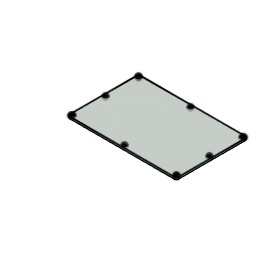
Lid - Compact (Autodesk Fusion 360 design; units mm, degrees)
Autodesk Fusion 360 part; units mm, degrees
sketch "Sketch1" plane through (0, 0, 123.8) normal (0, 0, 1) x (-1, 0, 0)
  line L0 (68.8, -91.5) -> (68.8, -99.5)
  line L1 (68.8, -99.5) -> (86.5, -99.5)
  arc A0 (86.5, -99.5) -> (89.5, -96.5) centre (86.5, -96.5) ccw
  line L2 (89.5, -96.5) -> (89.5, 14.2937)
  arc A1 (89.5, 14.2937) -> (86.5, 17.2937) centre (86.5, 14.2937) ccw
  line L3 (86.5, 17.2937) -> (-86.5, 17.2937)
  arc A2 (-86.5, 17.2937) -> (-89.5, 14.2937) centre (-86.5, 14.2937) ccw
  line L4 (-89.5, 14.2937) -> (-89.5, -96.5)
  arc A3 (-89.5, -96.5) -> (-86.5, -99.5) centre (-86.5, -96.5) ccw
  line L5 (-86.5, -99.5) -> (8.2, -99.5)
  line L6 (8.2, -99.5) -> (8.2, -91.5)
  line L7 (8.2, -91.5) -> (-71.5, -91.5)
  arc A4 (-81.5, -81.5) -> (-71.5, -91.5) centre (-71.5, -81.5) ccw
  line L8 (-81.5, -81.5) -> (-81.5, -0.7063)
  arc A5 (-71.5, 9.2937) -> (-81.5, -0.7063) centre (-71.5, -0.7063) ccw
  line L9 (-71.5, 9.2937) -> (71.5, 9.2937)
  arc A6 (81.5, -0.7063) -> (71.5, 9.2937) centre (71.5, -0.7063) ccw
  line L10 (81.5, -0.7063) -> (81.5, -81.5)
  arc A7 (71.5, -91.5) -> (81.5, -81.5) centre (71.5, -81.5) ccw
  line L11 (71.5, -91.5) -> (68.8, -91.5)
  circle A8 centre (-85.5, -95.5) radius 1.9
  circle A9 centre (85.5, 13.2937) radius 1.9
  circle A10 centre (85.5, -95.5) radius 1.9
  circle A11 centre (0, 13.2937) radius 1.9
  circle A12 centre (-85.5, -41.1031) radius 1.9
  circle A13 centre (-85.5, 13.2937) radius 1.9
  circle A14 centre (85.5, -41.1031) radius 1.9
  circle A15 centre (0, -95.5) radius 1.9
  line L12 (68.8, -99.5) -> (8.2, -99.5)
  constraint coincident L0.end L1.start
  constraint coincident L5.end L6.start
extrude "Extrude1" add sketch "Sketch1" along normal blind 3
sketch "Sketch2" plane through (0, 0, 126.8) normal (0, 0, 1) x (-1, 0, 0)
  circle A0 centre (-85.5, 13.2937) radius 1.9
  circle A1 centre (85.5, 13.2937) radius 1.9
  circle A2 centre (-85.5, -41.1031) radius 1.9
  circle A3 centre (85.5, -41.1031) radius 1.9
  circle A4 centre (0, 13.2937) radius 1.9
  circle A5 centre (-85.5, -95.5) radius 1.9
  circle A6 centre (0, -95.5) radius 1.9
  circle A7 centre (85.5, -95.5) radius 1.9
  arc A8 (86.5, -99.5) -> (89.5, -96.5) centre (86.5, -96.5) ccw
  line L0 (89.5, -96.5) -> (89.5, 14.2937)
  arc A9 (89.5, 14.2937) -> (86.5, 17.2937) centre (86.5, 14.2937) ccw
  line L1 (86.5, 17.2937) -> (-86.5, 17.2937)
  arc A10 (-86.5, 17.2937) -> (-89.5, 14.2937) centre (-86.5, 14.2937) ccw
  line L2 (-89.5, 14.2937) -> (-89.5, -96.5)
  arc A11 (-89.5, -96.5) -> (-86.5, -99.5) centre (-86.5, -96.5) ccw
  line L3 (-86.5, -99.5) -> (86.5, -99.5)
  circle A12 centre (85.5, -95.5) radius 2.3
  circle A13 centre (0, -95.5) radius 2.3
  circle A14 centre (-85.5, -95.5) radius 2.3
  circle A15 centre (-85.5, -41.1031) radius 2.3
  circle A16 centre (-85.5, 13.2937) radius 2.3
  circle A17 centre (0, 13.2937) radius 2.3
  circle A18 centre (85.5, 13.2937) radius 2.3
  circle A19 centre (85.5, -41.1031) radius 2.3
  line L4 (86.5, 17.0937) -> (-86.5, 17.0937)
  arc A20 (-86.5, 17.0937) -> (-89.3, 14.2937) centre (-86.5, 14.2937) ccw
  line L5 (-89.3, 14.2937) -> (-89.3, -96.5)
  arc A21 (-89.3, -96.5) -> (-86.5, -99.3) centre (-86.5, -96.5) ccw
  line L6 (-86.5, -99.3) -> (86.5, -99.3)
  arc A22 (86.5, -99.3) -> (89.3, -96.5) centre (86.5, -96.5) ccw
  line L7 (89.3, -96.5) -> (89.3, 14.2937)
  arc A23 (89.3, 14.2937) -> (86.5, 17.0937) centre (86.5, 14.2937) ccw
  dimension "d1290" = 4.6
  dimension "d1291" = 4.6
  dimension "d1292" = 4.6
  dimension "d1293" = 4.6
  dimension "d1294" = 4.6
  dimension "d1295" = 4.6
  dimension "d1296" = 4.6
  dimension "d1297" = 4.6
  dimension "d1300" = -0.2
  constraint concentric A7 A12
  constraint concentric A6 A13
  constraint concentric A5 A14
  constraint concentric A2 A15
  constraint concentric A0 A16
  constraint concentric A4 A17
  constraint concentric A1 A18
  constraint concentric A3 A19
  measures "d1290" diameter of A12
  measures "d1291" diameter of A13
  measures "d1292" diameter of A14
  measures "d1293" diameter of A15
  measures "d1294" diameter of A16
  measures "d1295" diameter of A17
  measures "d1296" diameter of A18
  measures "d1297" diameter of A19
extrude "Extrude3" cut sketch "Sketch2" against normal blind 3 contours A8 L0 A9 L1 A10 L2 A11 L3
extrude "Extrude2" cut sketch "Sketch2" against normal blind 3 contours A12 | A13 | A14 | A15 | A16 | A17 | A18
equation "d1291 = d1290"
equation "d1292 = d1290"
equation "d1293 = d1290"
equation "d1294 = d1290"
equation "d1295 = d1290"
equation "d1296 = d1290"
equation "d1297 = d1290"
